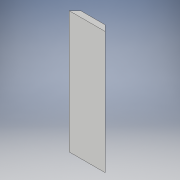
# Autodesk Inventor part: Fetch Charing Dock
Saved by Autodesk Inventor 2018 (Build 220112000, 112)
## iProperties
Created: 2020-01-05
Part Number: Fetch Charing Dock
Material: Generic
Document SubType Name: Modeling
Designer: roald_000
Density: 1 g/cm^3
Appearance: Default
Author: roald_000
Autodesk Inventor part; units mm, degrees
ref_plane "YZ Plane" through (0, 0, 0) normal (1, 0, 0) x (0, 1, 0)
ref_plane "XZ Plane" through (0, 0, 0) normal (0, 1, 0) x (-1, 0, 0)
ref_plane "XY Plane" through (0, 0, 0) normal (0, 0, 1) x (1, 0, 0)
sketch "Sketch2" plane through (0, 0, 0) normal (0, 1, 0) x (-1, 0, 0)
  line L0 (0, -70.71) -> (441.42, -70.71)
  line L1 (441.42, -70.71) -> (441.42, 0)
  line L2 (441.42, 0) -> (0, 0)
  line L3 (0, 0) -> (0, -70.71)
  dimension "d2" = 441.42
  dimension "d3" = 70.71
  constraints: 8 end point, 2 parallel, 1 coincident, 1 horizontal, 1 perpendicular
  measures "d2" distance between parallel lines of L1 L3
  measures "d3" distance between parallel lines of L2 L0
extrude "Extrusion1" add sketch "Sketch2" along normal blind 1500
sketch "Sketch3" plane through (0, 1500, 0) normal (0, 1, 0) x (1, 0, 0)
  line L0 (0, 70.71) -> (-441.42, 70.71) projected
  line L1 (-441.42, 0) -> (0, 0) projected
  line L2 (-370.71, 70.71) -> (-441.42, 0)
  line L3 (-70.71, 70.71) -> (0, 0)
  line L4 (-441.42, 70.71) -> (-441.42, 0) projected
  line L5 (-441.42, 70.71) -> (-441.42, 0)
  line L6 (-441.42, 70.71) -> (-370.71, 70.71)
  line L7 (0, 0) -> (0, 70.71)
  line L8 (-70.71, 70.71) -> (0, 70.71)
  dimension "d6" = 70.71
  dimension "d7" = 70.71
  constraints: 12 end point, 3 collinear, 2 point on line, 1 perpendicular
  measures "d6" distance of L0.end L2.start
  measures "d7" distance of L0.start L3.start
extrude "Extrusion2" cut sketch "Sketch3" against normal blind 1500 contours L7 L3 L0 | L2 L4 L0
body "Solid1"
